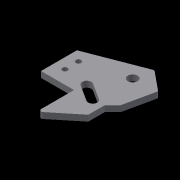
# Autodesk Inventor part: PelvisMountRight
Saved by Autodesk Inventor 2015 (Build 190159000, 159)
## iProperties
Created: 2014-12-04
Part Number: PelvisMountRight
Material: Generic
Document SubType Name: Modeling
Designer: Val
Density: 1 g/cm^3
Appearance: Default
Mass: 6.67837 g
Surface Area: 44.4409 cm^2
Volume: 6.67837 cm^3
Author: Val
Autodesk Inventor part; units mm, degrees
ref_plane "YZ Plane" through (0, 0, 0) normal (1, 0, 0) x (0, 1, 0)
ref_plane "XZ Plane" through (0, 0, 0) normal (0, 1, 0) x (-1, 0, 0)
ref_plane "XY Plane" through (0, 0, 0) normal (0, 0, 1) x (1, 0, 0)
sketch "Body" plane through (0, 0, 0) normal (0, 0, 1) x (1, 0, 0)
  circle A0 centre (-23.0092, 40.2765) radius 3.25
  circle A1 centre (-50.8524, 23.0069) radius 1.75
  circle A2 centre (-50.8524, 32.0069) radius 1.75
  line L0 (-16.8663, 15.4916) -> (-11.5626, 20.7945)
  line L1 (-16.8663, 4.4916) -> (-16.8663, 15.4916)
  line L2 (-35.8524, -10.9931) -> (-16.8663, 4.4916)
  arc A3 (-25.5002, 11.9918) -> (-22.2764, 17.0521) centre (-23.8883, 14.522) ccw
  line L3 (-25.5002, 11.9918) -> (-36.4643, 18.9767)
  line L4 (-22.2764, 17.0521) -> (-33.2405, 24.037)
  arc A4 (-33.2405, 24.037) -> (-36.4643, 18.9767) centre (-34.8524, 21.5069) ccw
  line L5 (-57.8524, 37.9418) -> (-20.5092, 52.2765)
  line L6 (-40.8524, 38.0069) -> (-60.8524, 38.0069) construction
  line L7 (-35.8524, 14.0069) -> (-35.8524, -10.9931)
  line L8 (-20.5092, 52.2765) -> (-7.101, 41.3151)
  line L9 (-7.101, 41.3151) -> (-11.5626, 20.7945)
  line L10 (-57.8524, 37.9418) -> (-57.8524, 14.0069)
  line L11 (-35.8524, 14.0069) -> (-57.8524, 14.0069)
  line L12 (-50.8524, 38.0069) -> (-50.8524, 23.0069) construction
  line L13 (-34.8524, 21.5069) -> (-23.8883, 14.522) construction
  point P0 (0, 0)
  dimension "d12" = 24
  dimension "d13" = 20
  dimension "d14" = 3.5
  dimension "d15" = 6
  dimension "d16" = 9
  dimension "d19" = 12
  dimension "d20" = 2.5
  dimension "d21" = 6.5
  dimension "d22" = 57.5
  dimension "d23" = 22
  dimension "d24" = 25
  dimension "d25" = 50.8
  dimension "d26" = 24.5
  dimension "d27" = 134.996
  dimension "d28" = 11
  dimension "d29" = 21
  dimension "d30" = 7.5
  dimension "d31" = 117
  dimension "d33" = 3
  dimension "d34" = 7.5
  dimension "d35" = 1
  dimension "d36" = 13
  dimension "d37" = 7
  dimension "d41" = 40
  dimension "d42" = 111
  constraints: 28 end point, 5 centre point, 4 point on circle, 4 tangent, 3 vertical, 2 horizontal, 2 parallel, 1 equal radius, 1 midpoint, 1 point on line, 1 other
  measures "d12" distance between parallel lines of L11 L6
  measures "d13" distance of L6.start L6.end
  measures "d14" diameter of A2
  measures "d15" distance from line of A2.centre L6
  measures "d16" distance of L12.end A2.centre
  measures "d19" vertical distance of A0.centre L5.end
  measures "d20" horizontal distance of L5.end A0.centre
  measures "d21" diameter of A0
  measures "d22" angle of L13 L7
  measures "d23" distance of L7.start L10.end
  measures "d24" distance of L7.start L2.start
  measures "d25" angle of L2 L7
  measures "d26" distance of L2.start L1.start
  measures "d27" angle of L0 L1
  measures "d28" distance of L1.start L0.start
  measures "d29" distance of L8.end L0.end
  measures "d30" distance of L0.start L0.end
  measures "d31" angle of L8 L9
  measures "d33" radius of A4
  measures "d34" vertical distance of L7.start L13.start
  measures "d35" horizontal distance of L7.start L13.start
  measures "d36" distance of L4.start L4.end
  measures "d37" distance between parallel lines of L10 L12
  measures "d41" distance of L5.start L5.end
  measures "d42" angle of L5 L10
extrude "BodyFeature" add sketch "Body" along normal blind 4
fillet "BodyFilletsFeature" radius 1.5 3 edges at (-35.8524, -10.9931, 2) (-20.5092, 52.2765, 2) (-7.101, 41.3151, 2)
